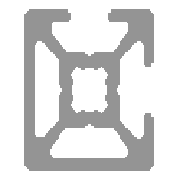
# Autodesk Inventor part: 3 842 992 924-25mm
Saved by Autodesk Inventor 2011 SP1 (Build 150282100, 282)
## iProperties
Created: 2011-02-10
Part Number: 3 842 992 924-25mm
Document SubType Name: Modeling
Designer: S. Wile
Density: 2.71 g/cm^3
Categories: <MemberInstance><Categories><Category DisplayName="Structural Shapes" InternalName="089c4875-fa83-4c05-b084-43b9cc11f5ed" Mnemonic="GRDR"><CategoryParameter DisplayName="Custom Base Point" InternalName="4f1d1b73-316d-484b-a3df-9cbabb16eb77" Mnemonic="shpBasePoint"/><CategoryParameter DisplayName="FG Authored" InternalName="9c666724-f362-4ea7-ac62-f6a007de5c69" Mnemonic="shpFGAuto"/><CategoryParameter DisplayName="Legacy Member ID" InternalName="340afe4f-75d7-48d3-ab7d-943f3c3da468" Mnemonic="LegacyMemberID"/><CategoryParameter DisplayName="Base Length" InternalName="42e34263-8f20-4d0e-ad48-bf1385b87c24" Mnemonic="shplen"/><CategoryParameter DisplayName="Distance of the Center of Gravity X-X" InternalName="26c9bdb8-9c79-4b4f-a92e-8e197583c9c4" Mnemonic="grcendistX"/><CategoryParameter DisplayName="Distance of the Center of Gravity Y-Y" InternalName="bcc4fb17-7af4-436a-8f8c-d0aa3b0248c5" Mnemonic="grcendistY"/><CategoryParameter DisplayName="Torsional Rigidity Modulus" InternalName="26c1ec35-5026-4c63-ad0a-751cf684a536" Mnemonic="torrigmod"/><CategoryParameter DisplayName="Torsional Section Modulus" InternalName="7c55a8dc-8844-49f9-a867-cc677b30ec9a" Mnemonic="torsecmod"/><CategoryParameter DisplayName="Coefficient of Shear Displacement" InternalName="de4c90c6-aaa8-468f-a335-6737b311b5d3" Mnemonic="shdispc"/><CategoryParameter DisplayName="Section Area" InternalName="1ff91680-64b0-4202-b9a3-7fd3f94bba3b" Mnemonic="secarea"/><CategoryParameter DisplayName="Moment of Inertia (x)" InternalName="4cd780bc-73d7-43ac-917a-579e5cbd684d" Mnemonic="inermomx"/><CategoryParameter DisplayName="Moment of Inertia (y)" InternalName="4b9f58ea-bced-460e-81ea-3d29ca5a49e3" Mnemonic="inermomy"/><CategoryParameter DisplayName="Section Module (x)" InternalName="72cfad18-cf51-4ed4-aaa7-c6b224f8419f" Mnemonic="secmodx"/><CategoryParameter DisplayName="Section Module (y)" InternalName="59eaa5e9-d227-48dc-b6c1-6920f96e0f95" Mnemonic="secmody"/><CategoryParameter DisplayName="Radius of Gyration (x)" InternalName="25778675-03e9-40c1-b6a8-4a9ed693320d" Mnemonic="gyrradx"/><CategoryParameter DisplayName="Radius of Gyration (y)" InternalName="bfa18ebe-1636-4dbe-8d42-b263e0b73184" Mnemonic="gyrrady"/><CategoryParameter DisplayName="Shape Thickness" InternalName="d109cf76-8eb4-42fc-9800-4409734adc67" Mnemonic="shpthick"/><CategoryParameter DisplayName="Second Shape Thickness" InternalName="9251a8e1-85fd-4e47-af99-afdb762317d9" Mnemonic="shpthick2"/><CategoryParameter DisplayName="Shape Width" InternalName="7c717d54-a18f-4666-b4d4-573cce22c62c" Mnemonic="shpwdth"/><CategoryParameter DisplayName="Shape Height" InternalName="50274e7d-5ac0-4796-92cb-c59e54983c67" Mnemonic="shpheig"/><CategoryParameter DisplayName="Mass per Length Unit" InternalName="0bb95a10-148f-4027-a459-38d7b056702a" Mnemonic="shpmass"/><CategoryParameter DisplayName="Section Designation" InternalName="5a64d034-428d-49c8-ba32-7619764de20f" Mnemonic="shpdes"/><Category DisplayName="Other" InternalName="f02205ff-2390-476f-921c-0b3185f88e84" Mnemonic="OTHSHP"><CategoryParameter DisplayName="Moment of Inertia (x)" InternalName="ec6737bc-264f-43ed-b0bd-f6d410c2718d" Mnemonic="inermomx"/><CategoryParameter DisplayName="Moment of Inertia (y)" InternalName="044c654e-f649-48ac-84cc-650a29ae31ca" Mnemonic="inermomy"/><CategoryParameter DisplayName="Section Module (x)" InternalName="cac70804-9d39-43bb-be17-56ea1f39a6c2" Mnemonic="secmodx"/><CategoryParameter DisplayName="Section Module (y)" InternalName="88b8bff9-a616-4028-93d5-ed4f79680d13" Mnemonic="secmody"/><CategoryParameter DisplayName="Section Area" InternalName="c46ecdf8-b6eb-4db9-8b25-30258930c1e3" Mnemonic="secarea"/><CategoryParameter DisplayName="Radius of Gyration (x)" InternalName="ee72c61e-565e-4fd6-b448-66e1e1abcb7e" Mnemonic="gyrradx"/><CategoryParameter DisplayName="Radius of Gyration (y)" InternalName="743e1dfe-1bba-408b-b985-cf752b207386" Mnemonic="gyrrady"/><CategoryParameter DisplayName="Shape Thickness" InternalName="12b1a788-9233-48fd-a933-2df8ff42b15f" Mnemonic="shpthick"/><CategoryParameter DisplayName="Mass per Length Unit" InternalName="2fd289d6-9394-4d2d-97e6-6659d7d4551d" Mnemonic="shpmass"/></Category></Category></Categories><FamilyTemplate Id="20x20-2SA"><FamilyTemplateParameters><FamilyTemplateParameter ObjectType="kUserParameterObject" ValueType="xs:double" Id="1" ObjectReferenceKey="G_L"/><FamilyTemplateParameter ObjectType="kUserParameterObject" ValueType="xs:double" Id="2" ObjectReferenceKey="G_OFFSET_END"/><FamilyTemplateParameter ObjectType="kUserParameterObject" ValueType="xs:double" Id="3" ObjectReferenceKey="G_OFFSET_START"/><FamilyTemplateParameter ObjectType="kUserParameterObject" ValueType="xs:double" Id="4" ObjectReferenceKey="Length"/><FamilyTemplateParameter ObjectType="kPropertyObject" ValueType="xs:string" Id="7" ObjectReferenceKey="{32853F0F-3444-11d1-9E93-0060B03C1CA6}" SubObjectId="52"/><FamilyTemplateParameter ObjectType="kPartComponentDefinitionObject" ValueType="xs:string" Id="8" SubObjectId="Material"/><FamilyTemplateParameter ObjectType="kPropertyObject" ValueType="xs:string" Id="9" ObjectReferenceKey="{32853F0F-3444-11d1-9E93-0060B03C1CA6}" SubObjectId="5"/><FamilyTemplateParameter ObjectType="kPropertyObject" ValueType="xs:string" Id="10" ObjectReferenceKey="{32853F0F-3444-11D1-9E93-0060B03C1CA6}" SubObjectId="55"/><FamilyTemplateParameter ObjectType="kiPartTableColumnObject" ValueType="xs:string" Id="21" ObjectReferenceKey="FILENAME"/><FamilyTemplateParameter ObjectType="kiPartTableColumnObject" ValueType="xs:string" Id="22" ObjectReferenceKey="MEMBER_REVISION"/></FamilyTemplateParameters></FamilyTemplate><CategoryParameterMap><ParamToTemplateMap><ParamToTemplate CategoryParameter="//CategoryParameter[@InternalName='9c666724-f362-4ea7-ac62-f6a007de5c69']" ConstantValue="1"/><ParamToTemplate CategoryParameter="//CategoryParameter[@InternalName='2675968c-4ce5-49e0-a4f5-552d29089031']" TemplateParameter="7"/><ParamToTemplate CategoryParameter="//CategoryParameter[@InternalName='8b46a4cc-9585-4fed-90c3-899f57e09a73']" TemplateParameter="21"/><ParamToTemplate CategoryParameter="//CategoryParameter[@InternalName='42e34263-8f20-4d0e-ad48-bf1385b87c24']" TemplateParameter="4"/><ParamToTemplate CategoryParameter="//CategoryParameter[@InternalName='818a152a-d3c3-49ca-80ee-df7d91421b8e']" TemplateParameter="8"/><ParamToTemplate CategoryParameter="//CategoryParameter[@InternalName='a65d44b9-392f-4f4f-857b-e4b3d54996fe']" TemplateParameter="22"/><ParamToTemplate CategoryParameter="//CategoryParameter[@InternalName='016b6077-bfbe-49bd-92c9-d8d59c39c941']" TemplateParameter="9"/></ParamToTemplateMap></CategoryParameterMap></MemberInstance>
Stock Number: 3 842 992 924
Description: PROFILE 20x20 2SA, -/-
Material: Aluminum-6061
Mass: 12.3805 g
Surface Area: 52.6277 cm^2
Volume: 4.56844 cm^3
Author: S. Wile
Autodesk Inventor part; units mm, degrees
ref_plane "YZ Plane" through (0, 0, 0) normal (1, 0, 0) x (0, 1, 0)
ref_plane "XZ Plane" through (0, 0, 0) normal (0, 1, 0) x (-1, 0, 0)
ref_plane "XY Plane" through (0, 0, 0) normal (0, 0, 1) x (1, 0, 0)
sketch "20x20-2SA" plane through (0, 0, 0) normal (0, 0, 1) x (1, 0, 0)
  arc A0 (98.9952, 77.0301) -> (99.4952, 77.5301) centre (98.9952, 77.5301) ccw
  line L0 (99.4952, 79.5301) -> (99.4952, 77.5301)
  arc A1 (99.9952, 80.0301) -> (99.4952, 79.5301) centre (99.9952, 79.5301) ccw
  line L1 (100.2952, 80.0301) -> (99.9952, 80.0301)
  arc A2 (100.4952, 79.8301) -> (100.2952, 80.0301) centre (100.2952, 79.8301) ccw
  line L2 (100.4952, 79.7301) -> (100.4952, 79.8301)
  arc A3 (100.4952, 79.7301) -> (100.6952, 79.5301) centre (100.6952, 79.7301) ccw
  line L3 (100.7952, 79.5301) -> (100.6952, 79.5301)
  arc A4 (100.9952, 79.3301) -> (100.7952, 79.5301) centre (100.7952, 79.3301) ccw
  line L4 (100.9952, 74.5301) -> (100.9952, 79.3301)
  arc A5 (99.4952, 73.0301) -> (100.9952, 74.5301) centre (99.4952, 74.5301) ccw
  line L5 (82.4952, 73.0301) -> (99.4952, 73.0301)
  arc A6 (80.9952, 74.5301) -> (82.4952, 73.0301) centre (82.4952, 74.5301) ccw
  line L6 (80.9952, 91.5301) -> (80.9952, 74.5301)
  arc A7 (82.4952, 93.0301) -> (80.9952, 91.5301) centre (82.4952, 91.5301) ccw
  line L7 (87.2452, 93.0301) -> (82.4952, 93.0301)
  arc A8 (87.4452, 92.8301) -> (87.2452, 93.0301) centre (87.2452, 92.8301) ccw
  line L8 (87.4452, 92.7301) -> (87.4452, 92.8301)
  arc A9 (87.4452, 92.7301) -> (87.6452, 92.5301) centre (87.6452, 92.7301) ccw
  line L9 (87.7952, 92.5301) -> (87.6452, 92.5301)
  arc A10 (87.9952, 92.3301) -> (87.7952, 92.5301) centre (87.7952, 92.3301) ccw
  line L10 (87.9952, 92.0301) -> (87.9952, 92.3301)
  arc A11 (87.4952, 91.5301) -> (87.9952, 92.0301) centre (87.4952, 92.0301) ccw
  line L11 (85.5452, 91.5301) -> (87.4952, 91.5301)
  arc A12 (85.5452, 91.5301) -> (85.0452, 91.0301) centre (85.5452, 91.0301) ccw
  line L12 (85.0452, 90.2979) -> (85.0452, 91.0301)
  arc A13 (85.0452, 90.2979) -> (85.1916, 89.9443) centre (85.5452, 90.2979) ccw
  line L13 (87.4594, 87.6765) -> (85.1916, 89.9443)
  arc A14 (87.4594, 87.6765) -> (87.8129, 87.5301) centre (87.8129, 88.0301) ccw
  line L14 (90.0916, 87.5301) -> (87.8129, 87.5301)
  arc A15 (90.1916, 87.5033) -> (90.0916, 87.5301) centre (90.0916, 87.3301) ccw
  line L15 (90.9452, 87.0682) -> (90.1916, 87.5033)
  arc A16 (90.9452, 87.0682) -> (91.1452, 87.0682) centre (91.0452, 87.2414) ccw
  line L16 (91.8988, 87.5033) -> (91.1452, 87.0682)
  arc A17 (91.9988, 87.5301) -> (91.8988, 87.5033) centre (91.9988, 87.3301) ccw
  line L17 (94.2774, 87.5301) -> (91.9988, 87.5301)
  arc A18 (94.2774, 87.5301) -> (94.6309, 87.6765) centre (94.2774, 88.0301) ccw
  arc A19 (92.9091, 80.0404) -> (93.9848, 81.1162) centre (90.9952, 83.0301) ccw
  line L18 (93.9848, 81.1162) -> (93.4405, 81.7719)
  arc A20 (93.4405, 81.7719) -> (93.4405, 84.2883) centre (90.9952, 83.0301) ccw
  line L19 (93.4405, 84.2883) -> (93.9848, 84.944)
  arc A21 (93.9848, 84.944) -> (92.9091, 86.0197) centre (90.9952, 83.0301) ccw
  line L20 (92.9091, 86.0197) -> (92.2533, 85.4754)
  arc A22 (92.2533, 85.4754) -> (89.737, 85.4754) centre (90.9952, 83.0301) ccw
  line L21 (89.737, 85.4754) -> (89.0813, 86.0197)
  arc A23 (89.0813, 86.0197) -> (88.0055, 84.944) centre (90.9952, 83.0301) ccw
  line L22 (88.0055, 84.944) -> (88.5499, 84.2883)
  arc A24 (88.5499, 84.2883) -> (88.5499, 81.7719) centre (90.9952, 83.0301) ccw
  line L23 (88.5499, 81.7719) -> (88.003, 81.1202)
  arc A25 (88.003, 81.1202) -> (89.0813, 80.0404) centre (90.9952, 83.0301) ccw
  line L24 (89.0813, 80.0404) -> (89.737, 80.5848)
  arc A26 (89.737, 80.5848) -> (92.2533, 80.5848) centre (90.9952, 83.0301) ccw
  line L25 (92.2533, 80.5848) -> (92.9091, 80.0404)
  arc A27 (86.4952, 83.9837) -> (86.522, 83.8837) centre (86.6952, 83.9837) ccw
  line L26 (86.4952, 83.9837) -> (86.4952, 86.2623)
  arc A28 (86.4952, 86.2623) -> (86.3487, 86.6159) centre (85.9952, 86.2623) ccw
  line L27 (86.3487, 86.6159) -> (84.0809, 88.8836)
  arc A29 (84.0809, 88.8836) -> (83.7274, 89.0301) centre (83.7274, 88.5301) ccw
  line L28 (83.7274, 89.0301) -> (82.9952, 89.0301)
  arc A30 (82.9952, 89.0301) -> (82.4952, 88.5301) centre (82.9952, 88.5301) ccw
  line L29 (82.4952, 88.5301) -> (82.4952, 77.5301)
  arc A31 (82.4952, 77.5301) -> (82.9952, 77.0301) centre (82.9952, 77.5301) ccw
  line L30 (82.9952, 77.0301) -> (83.7274, 77.0301)
  arc A32 (83.7274, 77.0301) -> (84.0809, 77.1765) centre (83.7274, 77.5301) ccw
  line L31 (84.0809, 77.1765) -> (86.3487, 79.4443)
  arc A33 (86.3487, 79.4443) -> (86.4952, 79.7979) centre (85.9952, 79.7979) ccw
  line L32 (86.4952, 79.7979) -> (86.4952, 82.0765)
  arc A34 (86.522, 82.1765) -> (86.4952, 82.0765) centre (86.6952, 82.0765) ccw
  line L33 (86.522, 82.1765) -> (86.957, 82.9301)
  arc A35 (86.957, 82.9301) -> (86.957, 83.1301) centre (86.7838, 83.0301) ccw
  line L34 (86.957, 83.1301) -> (86.522, 83.8837)
  arc A36 (96.4952, 74.5301) -> (96.9952, 75.0301) centre (96.4952, 75.0301) ccw
  line L35 (96.9952, 75.0301) -> (96.9952, 75.7623)
  arc A37 (96.9952, 75.7623) -> (96.8487, 76.1159) centre (96.4952, 75.7623) ccw
  line L36 (96.8487, 76.1159) -> (94.5809, 78.3836)
  arc A38 (94.5809, 78.3836) -> (94.2274, 78.5301) centre (94.2274, 78.0301) ccw
  line L37 (94.2274, 78.5301) -> (91.9488, 78.5301)
  arc A39 (91.8488, 78.5569) -> (91.9488, 78.5301) centre (91.9488, 78.7301) ccw
  line L38 (91.8488, 78.5569) -> (91.0952, 78.992)
  arc A40 (91.0952, 78.992) -> (90.8952, 78.992) centre (90.9952, 78.8188) ccw
  line L39 (90.8952, 78.992) -> (90.1416, 78.5569)
  arc A41 (90.0416, 78.5301) -> (90.1416, 78.5569) centre (90.0416, 78.7301) ccw
  line L40 (90.0416, 78.5301) -> (87.7629, 78.5301)
  arc A42 (87.7629, 78.5301) -> (87.4094, 78.3836) centre (87.7629, 78.0301) ccw
  line L41 (87.4094, 78.3836) -> (85.1416, 76.1159)
  arc A43 (85.1416, 76.1159) -> (84.9952, 75.7623) centre (85.4952, 75.7623) ccw
  line L42 (84.9952, 75.7623) -> (84.9952, 75.0301)
  arc A44 (84.9952, 75.0301) -> (85.4952, 74.5301) centre (85.4952, 75.0301) ccw
  line L43 (85.4952, 74.5301) -> (96.4952, 74.5301)
  line L44 (96.8987, 89.9443) -> (94.6309, 87.6765)
  arc A45 (96.8987, 89.9443) -> (97.0452, 90.2979) centre (96.5452, 90.2979) ccw
  line L45 (97.0452, 91.0301) -> (97.0452, 90.2979)
  arc A46 (97.0452, 91.0301) -> (96.5452, 91.5301) centre (96.5452, 91.0301) ccw
  line L46 (94.4952, 91.5301) -> (96.5452, 91.5301)
  arc A47 (93.9952, 92.0301) -> (94.4952, 91.5301) centre (94.4952, 92.0301) ccw
  line L47 (93.9952, 92.3301) -> (93.9952, 92.0301)
  arc A48 (94.1952, 92.5301) -> (93.9952, 92.3301) centre (94.1952, 92.3301) ccw
  line L48 (94.2952, 92.5301) -> (94.1952, 92.5301)
  arc A49 (94.2952, 92.5301) -> (94.4952, 92.7301) centre (94.2952, 92.7301) ccw
  line L49 (94.4952, 92.8301) -> (94.4952, 92.7301)
  arc A50 (94.6952, 93.0301) -> (94.4952, 92.8301) centre (94.6952, 92.8301) ccw
  line L50 (99.4952, 93.0301) -> (94.6952, 93.0301)
  arc A51 (100.9952, 91.5301) -> (99.4952, 93.0301) centre (99.4952, 91.5301) ccw
  line L51 (100.9952, 86.7301) -> (100.9952, 91.5301)
  arc A52 (100.7952, 86.5301) -> (100.9952, 86.7301) centre (100.7952, 86.7301) ccw
  line L52 (100.6952, 86.5301) -> (100.7952, 86.5301)
  arc A53 (100.6952, 86.5301) -> (100.4952, 86.3301) centre (100.6952, 86.3301) ccw
  line L53 (100.4952, 86.2301) -> (100.4952, 86.3301)
  arc A54 (100.2952, 86.0301) -> (100.4952, 86.2301) centre (100.2952, 86.2301) ccw
  line L54 (99.9952, 86.0301) -> (100.2952, 86.0301)
  arc A55 (99.4952, 86.5301) -> (99.9952, 86.0301) centre (99.9952, 86.5301) ccw
  line L55 (99.4952, 88.5301) -> (99.4952, 86.5301)
  arc A56 (99.4952, 88.5301) -> (98.9952, 89.0301) centre (98.9952, 88.5301) ccw
  line L56 (98.2629, 89.0301) -> (98.9952, 89.0301)
  arc A57 (98.2629, 89.0301) -> (97.9094, 88.8836) centre (98.2629, 88.5301) ccw
  line L57 (95.6416, 86.6159) -> (97.9094, 88.8836)
  arc A58 (95.6416, 86.6159) -> (95.4952, 86.2623) centre (95.9952, 86.2623) ccw
  line L58 (95.4952, 83.9837) -> (95.4952, 86.2623)
  arc A59 (95.4684, 83.8837) -> (95.4952, 83.9837) centre (95.2952, 83.9837) ccw
  line L59 (95.0333, 83.1301) -> (95.4684, 83.8837)
  arc A60 (95.0333, 83.1301) -> (95.0333, 82.9301) centre (95.2065, 83.0301) ccw
  line L60 (95.4684, 82.1765) -> (95.0333, 82.9301)
  arc A61 (95.4952, 82.0765) -> (95.4684, 82.1765) centre (95.2952, 82.0765) ccw
  line L61 (95.4952, 79.7979) -> (95.4952, 82.0765)
  arc A62 (95.4952, 79.7979) -> (95.6416, 79.4443) centre (95.9952, 79.7979) ccw
  line L62 (97.9094, 77.1765) -> (95.6416, 79.4443)
  arc A63 (97.9094, 77.1765) -> (98.2629, 77.0301) centre (98.2629, 77.5301) ccw
  line L63 (98.9952, 77.0301) -> (98.2629, 77.0301)
sketch "Sketch1" plane through (0, 0, 0) normal (0, 0, 1) x (1, 0, 0)
  arc A0 (8, -6) -> (8.5, -5.5) centre (8, -5.5) ccw
  line L0 (8.5, -3.5) -> (8.5, -5.5)
  arc A1 (9, -3) -> (8.5, -3.5) centre (9, -3.5) ccw
  line L1 (9.3, -3) -> (9, -3)
  arc A2 (9.5, -3.2) -> (9.3, -3) centre (9.3, -3.2) ccw
  line L2 (9.5, -3.3) -> (9.5, -3.2)
  arc A3 (9.5, -3.3) -> (9.7, -3.5) centre (9.7, -3.3) ccw
  line L3 (9.8, -3.5) -> (9.7, -3.5)
  arc A4 (10, -3.7) -> (9.8, -3.5) centre (9.8, -3.7) ccw
  line L4 (10, -8.5) -> (10, -3.7)
  arc A5 (8.5, -10) -> (10, -8.5) centre (8.5, -8.5) ccw
  line L5 (-8.5, -10) -> (8.5, -10)
  arc A6 (-10, -8.5) -> (-8.5, -10) centre (-8.5, -8.5) ccw
  line L6 (-10, 8.5) -> (-10, -8.5)
  arc A7 (-8.5, 10) -> (-10, 8.5) centre (-8.5, 8.5) ccw
  line L7 (-3.75, 10) -> (-8.5, 10)
  arc A8 (-3.55, 9.8) -> (-3.75, 10) centre (-3.75, 9.8) ccw
  line L8 (-3.55, 9.7) -> (-3.55, 9.8)
  arc A9 (-3.55, 9.7) -> (-3.35, 9.5) centre (-3.35, 9.7) ccw
  line L9 (-3.2, 9.5) -> (-3.35, 9.5)
  arc A10 (-3, 9.3) -> (-3.2, 9.5) centre (-3.2, 9.3) ccw
  line L10 (-3, 9) -> (-3, 9.3)
  arc A11 (-3.5, 8.5) -> (-3, 9) centre (-3.5, 9) ccw
  line L11 (-5.45, 8.5) -> (-3.5, 8.5)
  arc A12 (-5.45, 8.5) -> (-5.95, 8) centre (-5.45, 8) ccw
  line L12 (-5.95, 7.2678) -> (-5.95, 8)
  arc A13 (-5.95, 7.2678) -> (-5.8036, 6.9142) centre (-5.45, 7.2678) ccw
  line L13 (-3.5358, 4.6464) -> (-5.8036, 6.9142)
  arc A14 (-3.5358, 4.6464) -> (-3.1822, 4.5) centre (-3.1822, 5) ccw
  line L14 (-0.9036, 4.5) -> (-3.1822, 4.5)
  arc A15 (-0.8036, 4.4732) -> (-0.9036, 4.5) centre (-0.9036, 4.3) ccw
  line L15 (-0.05, 4.0381) -> (-0.8036, 4.4732)
  arc A16 (-0.05, 4.0381) -> (0.15, 4.0381) centre (0.05, 4.2113) ccw
  line L16 (0.9036, 4.4732) -> (0.15, 4.0381)
  arc A17 (1.0036, 4.5) -> (0.9036, 4.4732) centre (1.0036, 4.3) ccw
  line L17 (3.2822, 4.5) -> (1.0036, 4.5)
  arc A18 (3.2822, 4.5) -> (3.6358, 4.6464) centre (3.2822, 5) ccw
  arc A19 (1.9139, -2.9896) -> (2.9896, -1.9139) centre (0, 0) ccw
  line L18 (2.9896, -1.9139) -> (2.4453, -1.2582)
  arc A20 (2.4453, -1.2582) -> (2.4453, 1.2582) centre (0, 0) ccw
  line L19 (2.4453, 1.2582) -> (2.9896, 1.9139)
  arc A21 (2.9896, 1.9139) -> (1.9139, 2.9896) centre (0, 0) ccw
  line L20 (1.9139, 2.9896) -> (1.2582, 2.4453)
  arc A22 (1.2582, 2.4453) -> (-1.2582, 2.4453) centre (0, 0) ccw
  line L21 (-1.2582, 2.4453) -> (-1.9139, 2.9896)
  arc A23 (-1.9139, 2.9896) -> (-2.9896, 1.9139) centre (0, 0) ccw
  line L22 (-2.9896, 1.9139) -> (-2.4453, 1.2582)
  arc A24 (-2.4453, 1.2582) -> (-2.4453, -1.2582) centre (0, 0) ccw
  line L23 (-2.4453, -1.2582) -> (-2.9922, -1.9099)
  arc A25 (-2.9922, -1.9099) -> (-1.9139, -2.9896) centre (0, 0) ccw
  line L24 (-1.9139, -2.9896) -> (-1.2582, -2.4453)
  arc A26 (-1.2582, -2.4453) -> (1.2582, -2.4453) centre (0, 0) ccw
  line L25 (1.2582, -2.4453) -> (1.9139, -2.9896)
  arc A27 (-4.5, 0.9536) -> (-4.4732, 0.8536) centre (-4.3, 0.9536) ccw
  line L26 (-4.5, 0.9536) -> (-4.5, 3.2322)
  arc A28 (-4.5, 3.2322) -> (-4.6464, 3.5858) centre (-5, 3.2322) ccw
  line L27 (-4.6464, 3.5858) -> (-6.9142, 5.8536)
  arc A29 (-6.9142, 5.8536) -> (-7.2678, 6) centre (-7.2678, 5.5) ccw
  line L28 (-7.2678, 6) -> (-8, 6)
  arc A30 (-8, 6) -> (-8.5, 5.5) centre (-8, 5.5) ccw
  line L29 (-8.5, 5.5) -> (-8.5, -5.5)
  arc A31 (-8.5, -5.5) -> (-8, -6) centre (-8, -5.5) ccw
  line L30 (-8, -6) -> (-7.2678, -6)
  arc A32 (-7.2678, -6) -> (-6.9142, -5.8536) centre (-7.2678, -5.5) ccw
  line L31 (-6.9142, -5.8536) -> (-4.6464, -3.5858)
  arc A33 (-4.6464, -3.5858) -> (-4.5, -3.2322) centre (-5, -3.2322) ccw
  line L32 (-4.5, -3.2322) -> (-4.5, -0.9536)
  arc A34 (-4.4732, -0.8536) -> (-4.5, -0.9536) centre (-4.3, -0.9536) ccw
  line L33 (-4.4732, -0.8536) -> (-4.0381, -0.1)
  arc A35 (-4.0381, -0.1) -> (-4.0381, 0.1) centre (-4.2113, 0) ccw
  line L34 (-4.0381, 0.1) -> (-4.4732, 0.8536)
  arc A36 (5.5, -8.5) -> (6, -8) centre (5.5, -8) ccw
  line L35 (6, -8) -> (6, -7.2678)
  arc A37 (6, -7.2678) -> (5.8536, -6.9142) centre (5.5, -7.2678) ccw
  line L36 (5.8536, -6.9142) -> (3.5858, -4.6464)
  arc A38 (3.5858, -4.6464) -> (3.2322, -4.5) centre (3.2322, -5) ccw
  line L37 (3.2322, -4.5) -> (0.9536, -4.5)
  arc A39 (0.8536, -4.4732) -> (0.9536, -4.5) centre (0.9536, -4.3) ccw
  line L38 (0.8536, -4.4732) -> (0.1, -4.0381)
  arc A40 (0.1, -4.0381) -> (-0.1, -4.0381) centre (0, -4.2113) ccw
  line L39 (-0.1, -4.0381) -> (-0.8536, -4.4732)
  arc A41 (-0.9536, -4.5) -> (-0.8536, -4.4732) centre (-0.9536, -4.3) ccw
  line L40 (-0.9536, -4.5) -> (-3.2322, -4.5)
  arc A42 (-3.2322, -4.5) -> (-3.5858, -4.6464) centre (-3.2322, -5) ccw
  line L41 (-3.5858, -4.6464) -> (-5.8536, -6.9142)
  arc A43 (-5.8536, -6.9142) -> (-6, -7.2678) centre (-5.5, -7.2678) ccw
  line L42 (-6, -7.2678) -> (-6, -8)
  arc A44 (-6, -8) -> (-5.5, -8.5) centre (-5.5, -8) ccw
  line L43 (-5.5, -8.5) -> (5.5, -8.5)
  line L44 (5.9036, 6.9142) -> (3.6358, 4.6464)
  arc A45 (5.9036, 6.9142) -> (6.05, 7.2678) centre (5.55, 7.2678) ccw
  line L45 (6.05, 8) -> (6.05, 7.2678)
  arc A46 (6.05, 8) -> (5.55, 8.5) centre (5.55, 8) ccw
  line L46 (3.5, 8.5) -> (5.55, 8.5)
  arc A47 (3, 9) -> (3.5, 8.5) centre (3.5, 9) ccw
  line L47 (3, 9.3) -> (3, 9)
  arc A48 (3.2, 9.5) -> (3, 9.3) centre (3.2, 9.3) ccw
  line L48 (3.3, 9.5) -> (3.2, 9.5)
  arc A49 (3.3, 9.5) -> (3.5, 9.7) centre (3.3, 9.7) ccw
  line L49 (3.5, 9.8) -> (3.5, 9.7)
  arc A50 (3.7, 10) -> (3.5, 9.8) centre (3.7, 9.8) ccw
  line L50 (8.5, 10) -> (3.7, 10)
  arc A51 (10, 8.5) -> (8.5, 10) centre (8.5, 8.5) ccw
  line L51 (10, 3.7) -> (10, 8.5)
  arc A52 (9.8, 3.5) -> (10, 3.7) centre (9.8, 3.7) ccw
  line L52 (9.7, 3.5) -> (9.8, 3.5)
  arc A53 (9.7, 3.5) -> (9.5, 3.3) centre (9.7, 3.3) ccw
  line L53 (9.5, 3.2) -> (9.5, 3.3)
  arc A54 (9.3, 3) -> (9.5, 3.2) centre (9.3, 3.2) ccw
  line L54 (9, 3) -> (9.3, 3)
  arc A55 (8.5, 3.5) -> (9, 3) centre (9, 3.5) ccw
  line L55 (8.5, 5.5) -> (8.5, 3.5)
  arc A56 (8.5, 5.5) -> (8, 6) centre (8, 5.5) ccw
  line L56 (7.2678, 6) -> (8, 6)
  arc A57 (7.2678, 6) -> (6.9142, 5.8536) centre (7.2678, 5.5) ccw
  line L57 (4.6464, 3.5858) -> (6.9142, 5.8536)
  arc A58 (4.6464, 3.5858) -> (4.5, 3.2322) centre (5, 3.2322) ccw
  line L58 (4.5, 0.9536) -> (4.5, 3.2322)
  arc A59 (4.4732, 0.8536) -> (4.5, 0.9536) centre (4.3, 0.9536) ccw
  line L59 (4.0381, 0.1) -> (4.4732, 0.8536)
  arc A60 (4.0381, 0.1) -> (4.0381, -0.1) centre (4.2113, 0) ccw
  line L60 (4.4732, -0.8536) -> (4.0381, -0.1)
  arc A61 (4.5, -0.9536) -> (4.4732, -0.8536) centre (4.3, -0.9536) ccw
  line L61 (4.5, -3.2322) -> (4.5, -0.9536)
  arc A62 (4.5, -3.2322) -> (4.6464, -3.5858) centre (5, -3.2322) ccw
  line L62 (6.9142, -5.8536) -> (4.6464, -3.5858)
  arc A63 (6.9142, -5.8536) -> (7.2678, -6) centre (7.2678, -5.5) ccw
  line L63 (8, -6) -> (7.2678, -6)
  constraints: 1 other
extrude "Extrusion3" add sketch "Sketch1" along normal blind 30
body "Solid2"
